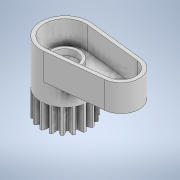
# Autodesk Inventor part: Klapphülle
Saved by Autodesk Inventor 2021 (Build 250183000, 183)
## iProperties
Created: 2021-01-08
Part Number: Klapphülle
Material: Generisch
Document SubType Name: Modeling
Designer: Jaro Machnow
Density: 1 g/cm^3
Appearance: Vorgabe
Author: Jaro Machnow
Autodesk Inventor part; units mm, degrees
ref_plane "YZ Plane" through (0, 0, 0) normal (1, 0, 0) x (0, 1, 0)
ref_plane "XZ Plane" through (0, 0, 0) normal (0, 1, 0) x (-1, 0, 0)
ref_plane "XY Plane" through (0, 0, 0) normal (0, 0, 1) x (1, 0, 0)
sketch "Skizze1" plane through (0, 0, 0) normal (0, 1, 0) x (-1, 0, 0)
  arc A0 (-2.1739, -19.8815) -> (-2.1739, 19.8815) centre (0, 0) ccw
  arc A1 (-47.6304, 14.9111) -> (-47.6304, -14.9111) centre (-46, 0) ccw
  line L0 (-2.1739, 19.8815) -> (-47.6304, 14.9111)
  line L1 (-2.1739, -19.8815) -> (-47.6304, -14.9111)
  line L2 (45.0235, 0) -> (-115.148, 0) construction
  dimension "Klapp_d_oben" = 40
  dimension "Klapp_d_unten" = 30
  dimension "Klapp_Abstand_oben_unten" = 46
  constraints: 6 end point, 4 point on circle, 4 tangent, 2 centre point, 2 horizontal, 1 coincident, 1 point on line
  measures "Klapp_d_oben" diameter of A0
  measures "Klapp_d_unten" diameter of A1
  measures "Klapp_Abstand_oben_unten" distance of A1.centre point (0, 0)
extrude "Extrusion1" add sketch "Skizze1" along normal blind 22
sketch "Skizze2" plane through (0, 22, 0) normal (0, 1, 0) x (1, 0, 0)
  arc A0 (47.6304, -14.9111) -> (47.6304, 14.9111) centre (46, 0) ccw projected
  line L0 (2.1739, -19.8815) -> (47.6304, -14.9111) projected
  arc A1 (47.6304, -14.9111) -> (47.6304, 14.9111) centre (46, 0) ccw projected
  line L1 (47.6304, 14.9111) -> (2.1739, 19.8815) projected
  arc A2 (2.1739, 19.8815) -> (2.1739, -19.8815) centre (0, 0) ccw projected
  circle A3 centre (46, 0) radius 5
  dimension "Klapp_Welle_Rad_d" = 10
  constraints: 1 centre point, 1 coincident
  measures "Klapp_Welle_Rad_d" diameter of A3
extrude "Extrusion2" [suppressed]
sketch "Skizze3" plane through (0, 0, 0) normal (0, -1, 0) x (1, 0, 0)
  circle A0 centre (0, 0) radius 9.5
  dimension "Klapp_Welle_Karosserie_d" = 19
  constraints: 1 centre point, 1 coincident
  measures "Klapp_Welle_Karosserie_d" diameter of A0
extrude "Extrusion3" [suppressed]
shell "Wandung1" thickness 3 removed faces 1 at (17.3261, 22, -4.9704)
sketch "Skizze7" plane through (0, 3, 0) normal (0, 1, 0) x (1, 0, 0)
  point P0 (0, 0)
sketch "Skizze9" plane through (0, 3, 0) normal (0, 1, 0) x (1, 0, 0)
  circle A0 centre (0, 0) radius 9.5
  circle A1 centre (0, 0) radius 12
  dimension "d25" = 19
  dimension "d26" = 24
  constraints: 2 centre point, 2 coincident
  measures "d25" diameter of A0
  measures "d26" diameter of A1
extrude "Extrusion6" add sketch "Skizze9" along normal blind 3
sketch "Skizze10" plane through (0, 3, 0) normal (0, 1, 0) x (1, 0, 0)
  circle A0 centre (0, 0) radius 9.5
  constraints: 1 centre point, 1 coincident
extrude "Extrusion7" cut sketch "Skizze10" against normal blind 2
sketch "Skizze11" plane through (0, 3, 0) normal (0, 1, 0) x (1, 0, 0)
  point P0 (0, 0)
sketch "Skizze12" plane through (0, 3, 0) normal (0, 1, 0) x (1, 0, 0)
  arc A0 (47.3043, -11.9289) -> (47.3043, 11.9289) centre (46, 0) ccw projected
  circle A1 centre (46, 0) radius 9.5
  circle A2 centre (46, 0) radius 12
  point P0 (0, 0)
  point P1 (47.3043, -11.9289)
  dimension "d31" = 19
  constraints: 2 centre point, 2 coincident, 1 concentric
  measures "d31" diameter of A1
extrude "Extrusion8" add sketch "Skizze12" along normal blind 3
sketch "Skizze13" plane through (46, 3, 0) normal (0, 1, 0) x (1, 0, 0)
  circle A0 centre (0, 0) radius 9.5
  point P0 (-46, 0)
  constraints: 1 centre point
extrude "Extrusion9" cut sketch "Skizze13" against normal blind 2
hole "Bohrung2" at (0, 3, 0) direction (0, -1, 0) diameter 11 end through all
sketch "Skizze15" plane through (0, 0, 0) normal (0, -1, 0) x (1, 0, 0)
  circle A0 centre (0, 0) radius 20
  circle A1 centre (0, 0) radius 12.5
  dimension "d44" = 25
  constraints: 2 centre point, 2 coincident
  measures "d44" diameter of A1
extrude "Extrusion10" add sketch "Skizze15" along normal blind 15
sketch "Skizze16" plane through (0, -15, 0) normal (0, -1, 0) x (1, 0, 0)
  arc A0 (-14.7826, -4.6609) -> (-14.3201, -5.9316) centre (0, 0) ccw
  arc A1 (-14.3201, -5.9316) -> (-17.7402, -9.235) centre (-5.261, -18.7329) ccw
  arc A2 (-17.7402, -9.235) -> (-16.8678, -10.746) centre (0, 0) ccw
  arc A3 (-16.8678, -10.746) -> (-12.297, -9.4358) centre (-18.8537, 4.8102) ccw
  arc A4 (-12.297, -9.4358) -> (-11.4278, -10.4716) centre (0, 0) ccw
  arc A5 (-11.4278, -10.4716) -> (-13.5118, -14.7455) centre (1.4633, -19.4025) ccw
  arc A6 (-13.5118, -14.7455) -> (-12.1752, -15.8671) centre (0, 0) ccw
  arc A7 (-8.3281, -13.0726) -> (-7.1571, -13.7487) centre (0, 0) ccw
  arc A8 (-12.1752, -15.8671) -> (-8.3281, -13.0726) centre (-19.3619, -1.9282) ccw
  arc A9 (-7.1571, 13.7487) -> (-8.3281, 13.0726) centre (0, 0) ccw
  arc A10 (-8.3281, 13.0726) -> (-12.1752, 15.8671) centre (-19.3619, 1.9282) ccw
  arc A11 (-12.1752, 15.8671) -> (-13.5118, 14.7455) centre (0, 0) ccw
  arc A12 (-11.4278, 10.4716) -> (-12.297, 9.4358) centre (0, 0) ccw
  arc A13 (-12.297, 9.4358) -> (-16.8678, 10.746) centre (-18.8537, -4.8102) ccw
  arc A14 (-14.3201, 5.9316) -> (-14.7826, 4.6609) centre (0, 0) ccw
  arc A15 (-16.8678, 10.746) -> (-17.7402, 9.235) centre (0, 0) ccw
  arc A16 (-17.7402, 9.235) -> (-14.3201, 5.9316) centre (-5.261, 18.7329) ccw
  arc A17 (-13.5118, 14.7455) -> (-11.4278, 10.4716) centre (1.4633, 19.4025) ccw
  arc A18 (-19.5259, -4.3288) -> (-14.7826, -4.6609) centre (-16.0715, 10.9685) ccw
  arc A19 (-19.8289, -2.6105) -> (-19.5259, -4.3288) centre (0, 0) ccw
  arc A20 (-15.4852, 0.6761) -> (-15.4852, -0.6761) centre (0, 0) ccw
  arc A21 (-15.4852, -0.6761) -> (-19.8289, -2.6105) centre (-11.3508, -15.8038) ccw
  arc A22 (-19.8289, 2.6105) -> (-15.4852, 0.6761) centre (-11.3508, 15.8038) ccw
  arc A23 (-14.7826, 4.6609) -> (-19.5259, 4.3288) centre (-16.0715, -10.9685) ccw
  arc A24 (-19.5259, 4.3288) -> (-19.8289, 2.6105) centre (0, 0) ccw
  arc A25 (-3.3548, -15.1326) -> (-2.0232, -15.3674) centre (0, 0) ccw
  arc A26 (-7.1571, -13.7487) -> (-7.6537, -18.4776) centre (8.0111, -17.732) ccw
  arc A27 (-7.6537, -18.4776) -> (-6.0141, -19.0743) centre (0, 0) ccw
  arc A28 (-6.0141, -19.0743) -> (-3.3548, -15.1326) centre (-17.5347, -8.434) ccw
  arc A29 (-2.0232, -15.3674) -> (-0.8724, -19.981) centre (13.5926, -13.9226) ccw
  arc A30 (0.8724, -19.981) -> (2.0232, -15.3674) centre (-13.5926, -13.9226) ccw
  arc A31 (-0.8724, -19.981) -> (0.8724, -19.981) centre (0, 0) ccw
  arc A32 (2.0232, -15.3674) -> (3.3548, -15.1326) centre (0, 0) ccw
  arc A33 (3.3548, -15.1326) -> (6.0141, -19.0743) centre (17.5347, -8.434) ccw
  arc A34 (6.0141, -19.0743) -> (7.6537, -18.4776) centre (0, 0) ccw
  arc A35 (7.6537, -18.4776) -> (7.1571, -13.7487) centre (-8.0111, -17.732) ccw
  arc A36 (7.1571, -13.7487) -> (8.3281, -13.0726) centre (0, 0) ccw
  arc A37 (8.3281, -13.0726) -> (12.1752, -15.8671) centre (19.3619, -1.9282) ccw
  arc A38 (11.4278, -10.4716) -> (12.297, -9.4358) centre (0, 0) ccw
  arc A39 (12.1752, -15.8671) -> (13.5118, -14.7455) centre (0, 0) ccw
  arc A40 (13.5118, -14.7455) -> (11.4278, -10.4716) centre (-1.4633, -19.4025) ccw
  arc A41 (14.3201, -5.9316) -> (14.7826, -4.6609) centre (0, 0) ccw
  arc A42 (12.297, -9.4358) -> (16.8678, -10.746) centre (18.8537, 4.8102) ccw
  arc A43 (17.7402, -9.235) -> (14.3201, -5.9316) centre (5.261, -18.7329) ccw
  arc A44 (16.8678, -10.746) -> (17.7402, -9.235) centre (0, 0) ccw
  arc A45 (19.5259, 4.3288) -> (14.7826, 4.6609) centre (16.0715, -10.9685) ccw
  arc A46 (19.8289, 2.6105) -> (19.5259, 4.3288) centre (0, 0) ccw
  arc A47 (15.4852, -0.6761) -> (15.4852, 0.6761) centre (0, 0) ccw
  arc A48 (15.4852, 0.6761) -> (19.8289, 2.6105) centre (11.3508, 15.8038) ccw
  arc A49 (19.8289, -2.6105) -> (15.4852, -0.6761) centre (11.3508, -15.8038) ccw
  arc A50 (14.7826, -4.6609) -> (19.5259, -4.3288) centre (16.0715, 10.9685) ccw
  arc A51 (19.5259, -4.3288) -> (19.8289, -2.6105) centre (0, 0) ccw
  arc A52 (14.7826, 4.6609) -> (14.3201, 5.9316) centre (0, 0) ccw
  arc A53 (8.3281, 13.0726) -> (7.1571, 13.7487) centre (0, 0) ccw
  arc A54 (12.297, 9.4358) -> (11.4278, 10.4716) centre (0, 0) ccw
  arc A55 (12.1752, 15.8671) -> (8.3281, 13.0726) centre (19.3619, 1.9282) ccw
  arc A56 (14.3201, 5.9316) -> (17.7402, 9.235) centre (5.261, 18.7329) ccw
  arc A57 (11.4278, 10.4716) -> (13.5118, 14.7455) centre (-1.4633, 19.4025) ccw
  arc A58 (13.5118, 14.7455) -> (12.1752, 15.8671) centre (0, 0) ccw
  arc A59 (16.8678, 10.746) -> (12.297, 9.4358) centre (18.8537, -4.8102) ccw
  arc A60 (17.7402, 9.235) -> (16.8678, 10.746) centre (0, 0) ccw
  arc A61 (-7.6537, 18.4776) -> (-7.1571, 13.7487) centre (8.0111, 17.732) ccw
  arc A62 (-6.0141, 19.0743) -> (-7.6537, 18.4776) centre (0, 0) ccw
  arc A63 (-3.3548, 15.1326) -> (-6.0141, 19.0743) centre (-17.5347, 8.434) ccw
  arc A64 (-2.0232, 15.3674) -> (-3.3548, 15.1326) centre (0, 0) ccw
  arc A65 (-0.8724, 19.981) -> (-2.0232, 15.3674) centre (13.5926, 13.9226) ccw
  arc A66 (3.3548, 15.1326) -> (2.0232, 15.3674) centre (0, 0) ccw
  arc A67 (2.0232, 15.3674) -> (0.8724, 19.981) centre (-13.5926, 13.9226) ccw
  arc A68 (6.0141, 19.0743) -> (3.3548, 15.1326) centre (17.5347, 8.434) ccw
  arc A69 (7.1571, 13.7487) -> (7.6537, 18.4776) centre (-8.0111, 17.732) ccw
  arc A70 (7.6537, 18.4776) -> (6.0141, 19.0743) centre (0, 0) ccw
  arc A71 (0.8724, 19.981) -> (-0.8724, 19.981) centre (0, 0) ccw
  circle A72 centre (0, 0) radius 12.5
  dimension "d47" = 25
  constraints: 144 point on circle, 73 centre point, 1 coincident
  measures "d47" diameter of A72
extrude "Extrusion11" add sketch "Skizze16" along normal blind 20
